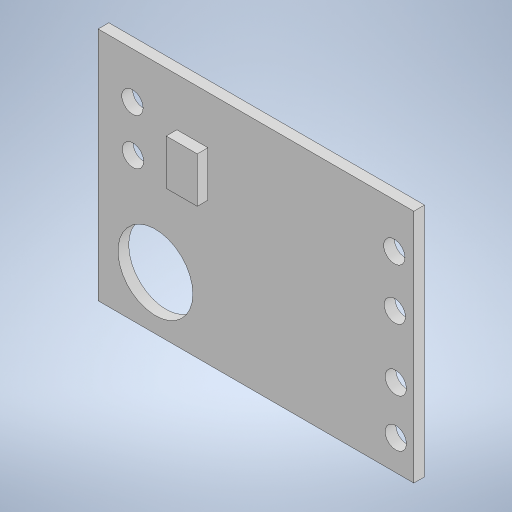
# Autodesk Inventor part: Laserový sensor vzdálenosti
Saved by Autodesk Inventor 2023 (Build 270158000, 158)
## iProperties
Created: 2023-01-20
Part Number: Laserový sensor vzdálenosti
Material: Všeobecné
Document SubType Name: Modeling
Designer: Kuba
Mass: 0.603978 g
Surface Area: 13.6031 cm^2
Volume: 0.603978 cm^3
Density: 1 g/cm^3
Appearance: Výchozí
Author: Kuba
Autodesk Inventor part; units mm, degrees
ref_plane "YZ Plane" through (0, 0, 0) normal (1, 0, 0) x (0, 1, 0)
ref_plane "XZ Plane" through (0, 0, 0) normal (0, 1, 0) x (-1, 0, 0)
ref_plane "XY Plane" through (0, 0, 0) normal (0, 0, 1) x (1, 0, 0)
sketch "Náčrt1" plane through (0, 0, 0) normal (0, 0, 1) x (1, 0, 0)
  line L0 (0, 0) -> (-14.75, 0) construction
  line L1 (-14.75, 0) -> (-14.75, -11) construction
  line L2 (-14.75, -11) -> (0, -11) construction
  line L3 (0, -11) -> (0, 0) construction
  line L4 (-14.75, -11) -> (14.75, -11)
  line L5 (14.75, -11) -> (14.75, 11)
  line L6 (14.75, 11) -> (-14.75, 11)
  line L7 (-14.75, 11) -> (-14.75, -11)
  dimension "d0" = 14.75
  dimension "d1" = 11
  dimension "d2" = 29.5
  dimension "d3" = 22
  constraints: 16 end point, 4 parallel, 2 horizontal, 2 perpendicular
  measures "d0" distance of L2.end L1.end
  measures "d1" distance of L1.end L0.end
  measures "d2" distance of L6.end L5.end
  measures "d3" distance of L5.end L4.end
extrude "Vysunutí1" add sketch "Náčrt1" along normal blind 1
sketch "Náčrt2" plane through (0, 0, 1) normal (0, 0, 1) x (1, 0, 0)
  point P0 (0, 0)
  point P1 (-9.3995, -6.0282)
hole "Díra1" at (-9.3995, -6.0282, 1) direction (0, 0, -1) diameter 7 end through all
sketch "Náčrt3" plane through (0, 0, 1) normal (0, 0, 1) x (1, 0, 0)
  point P0 (0, 0)
  point P1 (-11.4982, 2.4113)
hole "Díra2" at (-11.4982, 2.4113, 1) direction (0, 0, -1) diameter 2 end through all clearance for "Strojní šroub se zápustnou hlavou (82)" size "#1" standard "Ansi šroubové závity"
sketch "Náčrt4" plane through (0, 0, 1) normal (0, 0, 1) x (1, 0, 0)
  point P0 (0, 0)
  point P1 (-11.5429, 6.698)
hole "Díra3" at (-11.5429, 6.698, 1) direction (0, 0, -1) diameter 2 end through all clearance for "Strojní šroub se zápustnou hlavou (82)" size "#1" standard "Ansi šroubové závity"
sketch "Náčrt5" plane through (0, 0, 1) normal (0, 0, 1) x (1, 0, 0)
  point P0 (0, 0)
  point P1 (13.0611, -8.1715)
hole "Díra4" at (13.0611, -8.1715, 1) direction (0, 0, -1) diameter 2 end through all clearance for "Strojní šroub se zápustnou hlavou (82)" size "#1" standard "Ansi šroubové závity"
sketch "Náčrt6" plane through (0, 0, 1) normal (0, 0, 1) x (1, 0, 0)
  point P0 (0, 0)
  point P1 (13.0611, -3.7062)
hole "Díra5" at (13.0611, -3.7062, 1) direction (0, 0, -1) diameter 2 end through all clearance for "Strojní šroub se zápustnou hlavou (82)" size "#1" standard "Ansi šroubové závity"
sketch "Náčrt7" plane through (0, 0, 1) normal (0, 0, 1) x (1, 0, 0)
  point P0 (0, 0)
  point P1 (12.9718, 2.054)
hole "Díra6" at (12.9718, 2.054, 1) direction (0, 0, -1) diameter 2 end through all clearance for "Strojní šroub se zápustnou hlavou (82)" size "#1" standard "Ansi šroubové závity"
sketch "Náčrt8" plane through (0, 0, 1) normal (0, 0, 1) x (1, 0, 0)
  point P0 (0, 0)
  point P1 (12.9271, 6.8319)
hole "Díra7" at (12.9271, 6.8319, 1) direction (0, 0, -1) diameter 2 end through all clearance for "Strojní šroub se zápustnou hlavou (82)" size "#1" standard "Ansi šroubové závity"
sketch "Náčrt9" plane through (0, 0, 1) normal (0, 0, 1) x (1, 0, 0)
  line L0 (-7.3901, 6.5194) -> (-7.3901, 2.2773)
  line L1 (-7.3901, 2.2773) -> (-4.4876, 2.2773)
  line L2 (-4.4876, 2.2773) -> (-4.4876, 6.5194)
  line L3 (-4.4876, 6.5194) -> (-7.3901, 6.5194)
  point P0 (0, 0)
  constraints: 8 end point, 3 perpendicular, 1 vertical
extrude "Vysunutí2" add sketch "Náčrt9" along normal blind 1
